Autodesk Inventor part; units mm, degrees
(part 2 of 3)
  line L407 (-50.8399, 107.9096) -> (-50.0992, 107.9096) construction
  line L408 (-50.0992, 107.9096) -> (-49.4855, 107.2111) construction
  line L409 (-49.4855, 107.2111) -> (-49.4855, 106.0543) construction
  line L410 (-49.4855, 106.0543) -> (-49.4855, 105.3065) construction
  line L411 (-49.4855, 105.3065) -> (-49.7183, 104.6082) construction
  line L412 (-49.7183, 104.6082) -> (-49.9582, 104.2413) construction
  line L413 (-49.9582, 104.2413) -> (-50.0569, 104.1002) construction
  line L414 (-50.0569, 104.1002) -> (-50.1839, 104.0649) construction
  line L415 (-50.1839, 104.0649) -> (-50.2756, 104.0649) construction
  line L416 (-50.2756, 104.0649) -> (-50.4802, 104.0649) construction
  line L417 (-50.4802, 104.0649) -> (-50.6777, 104.2201) construction
  line L418 (-50.6777, 104.2201) -> (-50.6777, 104.4247) construction
  line L419 (-50.6777, 104.4247) -> (-50.6777, 104.5234) construction
  line L420 (-50.6777, 104.5234) -> (-50.6354, 104.6221) construction
  line L421 (-50.6354, 104.6221) -> (-50.5859, 104.721) construction
  line L422 (-50.5859, 104.721) -> (-50.3884, 105.116) construction
  line L423 (-50.3884, 105.116) -> (-50.2403, 105.5957) construction
  line L424 (-50.2403, 105.5957) -> (-50.2403, 106.0966) construction
  line L425 (-50.2403, 106.0966) -> (-50.2403, 106.7385) construction
  line L426 (-50.2403, 106.7385) -> (-50.4731, 107.0842) construction
  line L427 (-50.4731, 107.0842) -> (-50.8258, 107.0842) construction
  line L428 (-50.8258, 107.0842) -> (-51.2138, 107.0842) construction
  line L429 (-51.2138, 107.0842) -> (-51.3126, 106.7104) construction
  line L430 (-51.3126, 106.7104) -> (-51.4819, 105.8567) construction
  line L431 (-51.4819, 105.8567) -> (-51.6512, 104.9961) construction
  line L432 (-51.6512, 104.9961) -> (-51.8417, 104.1636) construction
  line L433 (-51.8417, 104.1636) -> (-52.8786, 104.1636) construction
  line L434 (-52.8786, 104.1636) -> (-53.5982, 104.1636) construction
  line L435 (-53.5982, 104.1636) -> (-54.2895, 104.8197) construction
  line L436 (-54.2895, 104.8197) -> (-54.2895, 106.0755) construction
  line L437 (-54.2895, 106.0755) -> (-54.2895, 106.7033) construction
  line L438 (-54.2895, 106.7033) -> (-54.0638, 107.2959) construction
  line L439 (-54.0638, 107.2959) -> (-53.9156, 107.5427) construction
  line L440 (-44.8705, 56.7364) -> (-43.6289, 56.7364)
  line L441 (-43.6289, 56.7364) -> (-43.6289, 58.4153)
  spline S53 degree 3 poles (-43.6289, 58.4153) (-43.6289, 58.6481) (-43.4878, 58.7892) (-43.2692, 58.7892) (-43.0505, 58.7892) (-42.9094, 58.6481) (-42.9094, 58.4153) knots 2 2 2 2 3 3 3 4 4 4 4
  line L442 (-43.6289, 58.4153) -> (-43.6289, 58.6481) construction
  line L443 (-43.6289, 58.6481) -> (-43.4878, 58.7892) construction
  line L444 (-43.4878, 58.7892) -> (-43.2692, 58.7892) construction
  line L445 (-43.2692, 58.7892) -> (-43.0505, 58.7892) construction
  line L446 (-43.0505, 58.7892) -> (-42.9094, 58.6481) construction
  line L447 (-42.9094, 58.6481) -> (-42.9094, 58.4153) construction
  line L448 (-42.9094, 58.4153) -> (-42.9094, 56.7364)
  line L449 (-42.9094, 56.7364) -> (-41.3997, 56.7364)
  spline S54 degree 3 poles (-41.3997, 56.7364) (-41.1881, 56.7364) (-41.0541, 56.5742) (-41.0541, 56.3484) (-41.0541, 56.1227) (-41.1881, 55.9604) (-41.3997, 55.9604) knots 6 6 6 6 7 7 7 8 8 8 8
  line L450 (-41.3997, 56.7364) -> (-41.1881, 56.7364) construction
  line L451 (-41.1881, 56.7364) -> (-41.0541, 56.5742) construction
  line L452 (-41.0541, 56.5742) -> (-41.0541, 56.3484) construction
  line L453 (-41.0541, 56.3484) -> (-41.0541, 56.1227) construction
  line L454 (-41.0541, 56.1227) -> (-41.1881, 55.9604) construction
  line L455 (-41.1881, 55.9604) -> (-41.3997, 55.9604) construction
  line L456 (-41.3997, 55.9604) -> (-45.4137, 55.9604)
  spline S55 degree 3 poles (-45.4137, 55.9604) (-45.6183, 55.9604) (-45.7452, 56.0874) (-45.7452, 56.3131) knots 9 9 9 9 10 10 10 10
  line L457 (-45.4137, 55.9604) -> (-45.6183, 55.9604) construction
  line L458 (-45.6183, 55.9604) -> (-45.7452, 56.0874) construction
  line L459 (-45.7452, 56.0874) -> (-45.7452, 56.3131) construction
  line L460 (-45.7452, 56.3131) -> (-45.7452, 59.0008)
  spline S56 degree 3 poles (-45.7452, 59.0008) (-45.7452, 59.2336) (-45.6112, 59.3748) (-45.3855, 59.3748) (-45.1668, 59.3748) (-45.0328, 59.2336) (-45.0328, 59.0079) knots 11 11 11 11 12 12 12 13 13 13 13
  line L461 (-45.7452, 59.0008) -> (-45.7452, 59.2336) construction
  line L462 (-45.7452, 59.2336) -> (-45.6112, 59.3748) construction
  line L463 (-45.6112, 59.3748) -> (-45.3855, 59.3748) construction
  line L464 (-45.3855, 59.3748) -> (-45.1668, 59.3748) construction
  line L465 (-45.1668, 59.3748) -> (-45.0328, 59.2336) construction
  line L466 (-45.0328, 59.2336) -> (-45.0328, 59.0079) construction
  line L467 (-45.0328, 59.0079) -> (-45.0328, 56.8775)
  spline S57 degree 3 poles (-45.0328, 56.8775) (-45.0328, 56.7787) (-44.9904, 56.7364) (-44.8705, 56.7364) knots 14 14 14 14 15 15 15 15
  line L468 (-45.0328, 56.8775) -> (-45.0328, 56.7787) construction
  line L469 (-45.0328, 56.7787) -> (-44.9904, 56.7364) construction
  line L470 (-44.9904, 56.7364) -> (-44.8705, 56.7364) construction
  spline S58 degree 3 poles (-43.4314, 59.714) (-44.8212, 59.714) (-45.8228, 60.7863) (-45.8228, 62.183) (-45.8228, 63.5798) (-44.8212, 64.6591) (-43.4314, 64.6591) (-42.0347, 64.6591) (-41.0259, 63.5798) (-41.0259, 62.183) (-41.0259, 60.7863) (-42.0347, 59.714) (-43.4314, 59.714) knots 0 0 0 0 1 1 1 2 2 2 3 3 3 4 4 4 4
  line L471 (-43.4314, 59.714) -> (-44.8212, 59.714) construction
  line L472 (-44.8212, 59.714) -> (-45.8228, 60.7863) construction
  line L473 (-45.8228, 60.7863) -> (-45.8228, 62.183) construction
  line L474 (-45.8228, 62.183) -> (-45.8228, 63.5798) construction
  line L475 (-45.8228, 63.5798) -> (-44.8212, 64.6591) construction
  line L476 (-44.8212, 64.6591) -> (-43.4314, 64.6591) construction
  line L477 (-43.4314, 64.6591) -> (-42.0347, 64.6591) construction
  line L478 (-42.0347, 64.6591) -> (-41.0259, 63.5798) construction
  line L479 (-41.0259, 63.5798) -> (-41.0259, 62.183) construction
  line L480 (-41.0259, 62.183) -> (-41.0259, 60.7863) construction
  line L481 (-41.0259, 60.7863) -> (-42.0347, 59.714) construction
  line L482 (-42.0347, 59.714) -> (-43.4314, 59.714) construction
  spline S59 degree 3 poles (-41.7878, 62.183) (-41.7878, 63.0507) (-42.4086, 63.8126) (-43.4244, 63.8126) (-44.4402, 63.8126) (-45.061, 63.0507) (-45.061, 62.183) (-45.061, 61.3224) (-44.4402, 60.5606) (-43.4244, 60.5606) (-42.4086, 60.5606) (-41.7878, 61.3224) (-41.7878, 62.183) knots 0 0 0 0 1 1 1 2 2 2 3 3 3 4 4 4 4
  line L483 (-41.7878, 62.183) -> (-41.7878, 63.0507) construction
  line L484 (-41.7878, 63.0507) -> (-42.4086, 63.8126) construction
  line L485 (-42.4086, 63.8126) -> (-43.4244, 63.8126) construction
  line L486 (-43.4244, 63.8126) -> (-44.4402, 63.8126) construction
  line L487 (-44.4402, 63.8126) -> (-45.061, 63.0507) construction
  line L488 (-45.061, 63.0507) -> (-45.061, 62.183) construction
  line L489 (-45.061, 62.183) -> (-45.061, 61.3224) construction
  line L490 (-45.061, 61.3224) -> (-44.4402, 60.5606) construction
  line L491 (-44.4402, 60.5606) -> (-43.4244, 60.5606) construction
  line L492 (-43.4244, 60.5606) -> (-42.4086, 60.5606) construction
  line L493 (-42.4086, 60.5606) -> (-41.7878, 61.3224) construction
  line L494 (-41.7878, 61.3224) -> (-41.7878, 62.183) construction
  line L495 (-42.8247, 68.1872) -> (-41.703, 69.3087)
  spline S60 degree 3 poles (-41.703, 69.3087) (-41.6184, 69.4005) (-41.5337, 69.4429) (-41.4279, 69.4429) (-41.2445, 69.4429) (-41.0541, 69.2736) (-41.0541, 69.0477) (-41.0541, 68.9208) (-41.1105, 68.8362) (-41.2023, 68.7515) knots 1 1 1 1 2 2 2 3 3 3 4 4 4 4
  line L496 (-41.703, 69.3087) -> (-41.6184, 69.4005) construction
  line L497 (-41.6184, 69.4005) -> (-41.5337, 69.4429) construction
  line L498 (-41.5337, 69.4429) -> (-41.4279, 69.4429) construction
  line L499 (-41.4279, 69.4429) -> (-41.2445, 69.4429) construction
  line L500 (-41.2445, 69.4429) -> (-41.0541, 69.2736) construction
  line L501 (-41.0541, 69.2736) -> (-41.0541, 69.0477) construction
  line L502 (-41.0541, 69.0477) -> (-41.0541, 68.9208) construction
  line L503 (-41.0541, 68.9208) -> (-41.1105, 68.8362) construction
  line L504 (-41.1105, 68.8362) -> (-41.2023, 68.7515) construction
  line L505 (-41.2023, 68.7515) -> (-42.719, 67.2983)
  line L506 (-42.719, 67.2983) -> (-42.719, 66.5083)
  line L507 (-42.719, 66.5083) -> (-41.3997, 66.5083)
  spline S61 degree 3 poles (-41.3997, 66.5083) (-41.1881, 66.5083) (-41.0541, 66.346) (-41.0541, 66.1203) (-41.0541, 65.8945) (-41.1881, 65.7323) (-41.3997, 65.7323) knots 7 7 7 7 8 8 8 9 9 9 9
  line L508 (-41.3997, 66.5083) -> (-41.1881, 66.5083) construction
  line L509 (-41.1881, 66.5083) -> (-41.0541, 66.346) construction
  line L510 (-41.0541, 66.346) -> (-41.0541, 66.1203) construction
  line L511 (-41.0541, 66.1203) -> (-41.0541, 65.8945) construction
  line L512 (-41.0541, 65.8945) -> (-41.1881, 65.7323) construction
  line L513 (-41.1881, 65.7323) -> (-41.3997, 65.7323) construction
  line L514 (-41.3997, 65.7323) -> (-45.4137, 65.7323)
  spline S62 degree 3 poles (-45.4137, 65.7323) (-45.6183, 65.7323) (-45.7452, 65.8592) (-45.7452, 66.085) knots 10 10 10 10 11 11 11 11
  line L515 (-45.4137, 65.7323) -> (-45.6183, 65.7323) construction
  line L516 (-45.6183, 65.7323) -> (-45.7452, 65.8592) construction
  line L517 (-45.7452, 65.8592) -> (-45.7452, 66.085) construction
  line L518 (-45.7452, 66.085) -> (-45.7452, 67.5381)
  spline S63 degree 3 poles (-45.7452, 67.5381) (-45.7452, 68.8362) (-45.0398, 69.3793) (-44.278, 69.3793) (-43.7065, 69.3793) (-43.0153, 69.0266) (-42.8247, 68.1872) knots 12 12 12 12 13 13 13 14 14 14 14
  line L519 (-45.7452, 67.5381) -> (-45.7452, 68.8362) construction
  line L520 (-45.7452, 68.8362) -> (-45.0398, 69.3793) construction
  line L521 (-45.0398, 69.3793) -> (-44.278, 69.3793) construction
  line L522 (-44.278, 69.3793) -> (-43.7065, 69.3793) construction
  line L523 (-43.7065, 69.3793) -> (-43.0153, 69.0266) construction
  line L524 (-43.0153, 69.0266) -> (-42.8247, 68.1872) construction
  spline S64 degree 3 poles (-43.4173, 67.4818) (-43.4173, 68.2576) (-43.7841, 68.5329) (-44.2285, 68.5329) (-44.666, 68.5329) (-45.0328, 68.2576) (-45.0328, 67.4818) knots 0 0 0 0 1 1 1 2 2 2 2
  line L525 (-43.4173, 67.4818) -> (-43.4173, 68.2576) construction
  line L526 (-43.4173, 68.2576) -> (-43.7841, 68.5329) construction
  line L527 (-43.7841, 68.5329) -> (-44.2285, 68.5329) construction
  line L528 (-44.2285, 68.5329) -> (-44.666, 68.5329) construction
  line L529 (-44.666, 68.5329) -> (-45.0328, 68.2576) construction
  line L530 (-45.0328, 68.2576) -> (-45.0328, 67.4818) construction
  line L531 (-45.0328, 67.4818) -> (-45.0328, 66.6493)
  spline S65 degree 3 poles (-45.0328, 66.6493) (-45.0328, 66.5506) (-44.9904, 66.5083) (-44.8705, 66.5083) knots 3 3 3 3 4 4 4 4
  line L532 (-45.0328, 66.6493) -> (-45.0328, 66.5506) construction
  line L533 (-45.0328, 66.5506) -> (-44.9904, 66.5083) construction
  line L534 (-44.9904, 66.5083) -> (-44.8705, 66.5083) construction
  line L535 (-44.8705, 66.5083) -> (-43.4173, 66.5083)
  line L536 (-43.4173, 66.5083) -> (-43.4173, 67.4818)
  line L537 (-44.546, 74.2405) -> (-43.0575, 73.2248)
  spline S66 degree 3 poles (-43.0575, 73.2248) (-42.8459, 73.0837) (-42.7613, 72.9707) (-42.7613, 72.7803) (-42.7613, 72.5969) (-42.8459, 72.4911) (-43.0575, 72.343) knots 1 1 1 1 2 2 2 3 3 3 3
  line L538 (-43.0575, 73.2248) -> (-42.8459, 73.0837) construction
  line L539 (-42.8459, 73.0837) -> (-42.7613, 72.9707) construction
  line L540 (-42.7613, 72.9707) -> (-42.7613, 72.7803) construction
  line L541 (-42.7613, 72.7803) -> (-42.7613, 72.5969) construction
  line L542 (-42.7613, 72.5969) -> (-42.8459, 72.4911) construction
  line L543 (-42.8459, 72.4911) -> (-43.0575, 72.343) construction
  line L544 (-43.0575, 72.343) -> (-44.546, 71.327)
  line L545 (-44.546, 71.327) -> (-44.546, 71.306)
  line L546 (-44.546, 71.306) -> (-41.3997, 71.306)
  spline S67 degree 3 poles (-41.3997, 71.306) (-41.1881, 71.306) (-41.0541, 71.1437) (-41.0541, 70.9179) (-41.0541, 70.6923) (-41.1881, 70.53) (-41.3997, 70.53) knots 6 6 6 6 7 7 7 8 8 8 8
  line L547 (-41.3997, 71.306) -> (-41.1881, 71.306) construction
  line L548 (-41.1881, 71.306) -> (-41.0541, 71.1437) construction
  line L549 (-41.0541, 71.1437) -> (-41.0541, 70.9179) construction
  line L550 (-41.0541, 70.9179) -> (-41.0541, 70.6923) construction
  line L551 (-41.0541, 70.6923) -> (-41.1881, 70.53) construction
  line L552 (-41.1881, 70.53) -> (-41.3997, 70.53) construction
  line L553 (-41.3997, 70.53) -> (-45.3361, 70.53)
  spline S68 degree 3 poles (-45.3361, 70.53) (-45.6112, 70.53) (-45.7876, 70.7274) (-45.7876, 70.9885) knots 9 9 9 9 10 10 10 10
  line L554 (-45.3361, 70.53) -> (-45.6112, 70.53) construction
  line L555 (-45.6112, 70.53) -> (-45.7876, 70.7274) construction
  line L556 (-45.7876, 70.7274) -> (-45.7876, 70.9885) construction
  line L557 (-45.7876, 70.9885) -> (-45.7876, 71.0449)
  spline S69 degree 3 poles (-45.7876, 71.0449) (-45.7876, 71.3131) (-45.6253, 71.4822) (-45.4137, 71.6233) knots 11 11 11 11 12 12 12 12
  line L558 (-45.7876, 71.0449) -> (-45.7876, 71.3131) construction
  line L559 (-45.7876, 71.3131) -> (-45.6253, 71.4822) construction
  line L560 (-45.6253, 71.4822) -> (-45.4137, 71.6233) construction
  line L561 (-45.4137, 71.6233) -> (-43.6925, 72.8015)
  line L562 (-43.6925, 72.8015) -> (-43.6925, 72.8086)
  line L563 (-43.6925, 72.8086) -> (-45.4208, 73.9796)
  spline S70 degree 3 poles (-45.4208, 73.9796) (-45.6253, 74.1206) (-45.7876, 74.2547) (-45.7876, 74.5227) knots 15 15 15 15 16 16 16 16
  line L564 (-45.4208, 73.9796) -> (-45.6253, 74.1206) construction
  line L565 (-45.6253, 74.1206) -> (-45.7876, 74.2547) construction
  line L566 (-45.7876, 74.2547) -> (-45.7876, 74.5227) construction
  line L567 (-45.7876, 74.5227) -> (-45.7876, 74.5792)
  spline S71 degree 3 poles (-45.7876, 74.5792) (-45.7876, 74.8331) (-45.6112, 75.0307) (-45.3361, 75.0307) knots 17 17 17 17 18 18 18 18
  line L568 (-45.7876, 74.5792) -> (-45.7876, 74.8331) construction
  line L569 (-45.7876, 74.8331) -> (-45.6112, 75.0307) construction
  line L570 (-45.6112, 75.0307) -> (-45.3361, 75.0307) construction
  line L571 (-45.3361, 75.0307) -> (-41.3997, 75.0307)
  spline S72 degree 3 poles (-41.3997, 75.0307) (-41.1881, 75.0307) (-41.0541, 74.8684) (-41.0541, 74.6426) (-41.0541, 74.4169) (-41.1881, 74.2547) (-41.3997, 74.2547) knots 19 19 19 19 20 20 20 21 21 21 21
  line L572 (-41.3997, 75.0307) -> (-41.1881, 75.0307) construction
  line L573 (-41.1881, 75.0307) -> (-41.0541, 74.8684) construction
  line L574 (-41.0541, 74.8684) -> (-41.0541, 74.6426) construction
  line L575 (-41.0541, 74.6426) -> (-41.0541, 74.4169) construction
  line L576 (-41.0541, 74.4169) -> (-41.1881, 74.2547) construction
  line L577 (-41.1881, 74.2547) -> (-41.3997, 74.2547) construction
  line L578 (-41.3997, 74.2547) -> (-44.546, 74.2547)
  line L579 (-44.546, 74.2547) -> (-44.546, 74.2405)
  spline S73 degree 3 poles (-41.7666, 78.3612) (-41.7666, 79.116) (-42.2815, 79.5887) (-43.0858, 79.5887) knots 0 0 0 0 1 1 1 1
  line L580 (-41.7666, 78.3612) -> (-41.7666, 79.116) construction
  line L581 (-41.7666, 79.116) -> (-42.2815, 79.5887) construction
  line L582 (-42.2815, 79.5887) -> (-43.0858, 79.5887) construction
  line L583 (-43.0858, 79.5887) -> (-45.449, 79.5887)
  spline S74 degree 3 poles (-45.449, 79.5887) (-45.6536, 79.5887) (-45.7947, 79.7508) (-45.7947, 79.9766) (-45.7947, 80.2023) (-45.6536, 80.3645) (-45.449, 80.3645) knots 2 2 2 2 3 3 3 4 4 4 4
  line L584 (-45.449, 79.5887) -> (-45.6536, 79.5887) construction
  line L585 (-45.6536, 79.5887) -> (-45.7947, 79.7508) construction
  line L586 (-45.7947, 79.7508) -> (-45.7947, 79.9766) construction
  line L587 (-45.7947, 79.9766) -> (-45.7947, 80.2023) construction
  line L588 (-45.7947, 80.2023) -> (-45.6536, 80.3645) construction
  line L589 (-45.6536, 80.3645) -> (-45.449, 80.3645) construction
  line L590 (-45.449, 80.3645) -> (-43.0434, 80.3645)
  spline S75 degree 3 poles (-43.0434, 80.3645) (-41.8723, 80.3645) (-41.0118, 79.6168) (-41.0118, 78.3612) (-41.0118, 77.0984) (-41.8723, 76.3577) (-43.0434, 76.3577) knots 5 5 5 5 6 6 6 7 7 7 7
  line L591 (-43.0434, 80.3645) -> (-41.8723, 80.3645) construction
  line L592 (-41.8723, 80.3645) -> (-41.0118, 79.6168) construction
  line L593 (-41.0118, 79.6168) -> (-41.0118, 78.3612) construction
  line L594 (-41.0118, 78.3612) -> (-41.0118, 77.0984) construction
  line L595 (-41.0118, 77.0984) -> (-41.8723, 76.3577) construction
  line L596 (-41.8723, 76.3577) -> (-43.0434, 76.3577) construction
  line L597 (-43.0434, 76.3577) -> (-45.449, 76.3577)
  spline S76 degree 3 poles (-45.449, 76.3577) (-45.6536, 76.3577) (-45.7947, 76.52) (-45.7947, 76.7456) (-45.7947, 76.9715) (-45.6536, 77.1337) (-45.449, 77.1337) knots 8 8 8 8 9 9 9 10 10 10 10
  line L598 (-45.449, 76.3577) -> (-45.6536, 76.3577) construction
  line L599 (-45.6536, 76.3577) -> (-45.7947, 76.52) construction
  line L600 (-45.7947, 76.52) -> (-45.7947, 76.7456) construction
  line L601 (-45.7947, 76.7456) -> (-45.7947, 76.9715) construction
  line L602 (-45.7947, 76.9715) -> (-45.6536, 77.1337) construction
  line L603 (-45.6536, 77.1337) -> (-45.449, 77.1337) construction
  line L604 (-45.449, 77.1337) -> (-43.0858, 77.1337)
  spline S77 degree 3 poles (-43.0858, 77.1337) (-42.2886, 77.1337) (-41.7666, 77.5993) (-41.7666, 78.3612) knots 11 11 11 11 12 12 12 12
  line L605 (-43.0858, 77.1337) -> (-42.2886, 77.1337) construction
  line L606 (-42.2886, 77.1337) -> (-41.7666, 77.5993) construction
  line L607 (-41.7666, 77.5993) -> (-41.7666, 78.3612) construction
  spline S78 degree 3 poles (-45.7876, 82.0797) (-45.7876, 82.3055) (-45.6536, 82.4678) (-45.449, 82.4678) knots 0 0 0 0 1 1 1 1
  line L608 (-45.7876, 82.0797) -> (-45.7876, 82.3055) construction
  line L609 (-45.7876, 82.3055) -> (-45.6536, 82.4678) construction
  line L610 (-45.6536, 82.4678) -> (-45.449, 82.4678) construction
  line L611 (-45.449, 82.4678) -> (-41.9853, 82.4678)
  spline S79 degree 3 poles (-41.9853, 82.4678) (-41.8582, 82.4678) (-41.8229, 82.51) (-41.8229, 82.6088) knots 2 2 2 2 3 3 3 3
  line L612 (-41.9853, 82.4678) -> (-41.8582, 82.4678) construction
  line L613 (-41.8582, 82.4678) -> (-41.8229, 82.51) construction
  line L614 (-41.8229, 82.51) -> (-41.8229, 82.6088) construction
  line L615 (-41.8229, 82.6088) -> (-41.8229, 84.6687)
  spline S80 degree 3 poles (-41.8229, 84.6687) (-41.8229, 84.9014) (-41.6889, 85.0425) (-41.4632, 85.0425) (-41.2374, 85.0425) (-41.1034, 84.9014) (-41.1034, 84.6687) knots 4 4 4 4 5 5 5 6 6 6 6
  line L616 (-41.8229, 84.6687) -> (-41.8229, 84.9014) construction
  line L617 (-41.8229, 84.9014) -> (-41.6889, 85.0425) construction
  line L618 (-41.6889, 85.0425) -> (-41.4632, 85.0425) construction
  line L619 (-41.4632, 85.0425) -> (-41.2374, 85.0425) construction
  line L620 (-41.2374, 85.0425) -> (-41.1034, 84.9014) construction
  line L621 (-41.1034, 84.9014) -> (-41.1034, 84.6687) construction
  line L622 (-41.1034, 84.6687) -> (-41.1034, 82.0726)
  spline S81 degree 3 poles (-41.1034, 82.0726) (-41.1034, 81.8399) (-41.2303, 81.6918) (-41.4632, 81.6918) knots 7 7 7 7 8 8 8 8
  line L623 (-41.1034, 82.0726) -> (-41.1034, 81.8399) construction
  line L624 (-41.1034, 81.8399) -> (-41.2303, 81.6918) construction
  line L625 (-41.2303, 81.6918) -> (-41.4632, 81.6918) construction
  line L626 (-41.4632, 81.6918) -> (-45.449, 81.6918)
  spline S82 degree 3 poles (-45.449, 81.6918) (-45.6536, 81.6918) (-45.7876, 81.854) (-45.7876, 82.0797) knots 9 9 9 9 10 10 10 10
  line L627 (-45.449, 81.6918) -> (-45.6536, 81.6918) construction
  line L628 (-45.6536, 81.6918) -> (-45.7876, 81.854) construction
  line L629 (-45.7876, 81.854) -> (-45.7876, 82.0797) construction
  line L630 (-42.2392, 86.6162) -> (-41.3433, 86.2495)
  spline S83 degree 3 poles (-41.3433, 86.2495) (-41.1528, 86.1718) (-41.0541, 86.0519) (-41.0541, 85.8684) (-41.0541, 85.6428) (-41.2023, 85.4876) (-41.4067, 85.4734) knots 1 1 1 1 2 2 2 3 3 3 3
  line L631 (-41.3433, 86.2495) -> (-41.1528, 86.1718) construction
  line L632 (-41.1528, 86.1718) -> (-41.0541, 86.0519) construction
  line L633 (-41.0541, 86.0519) -> (-41.0541, 85.8684) construction
  line L634 (-41.0541, 85.8684) -> (-41.0541, 85.6428) construction
  line L635 (-41.0541, 85.6428) -> (-41.2023, 85.4876) construction
  line L636 (-41.2023, 85.4876) -> (-41.4067, 85.4734) construction
  spline S84 degree 3 poles (-41.4067, 85.4734) (-41.4986, 85.4664) (-41.5831, 85.4946) (-41.6818, 85.537) knots 3 3 3 3 4 4 4 4
  line L637 (-41.4067, 85.4734) -> (-41.4986, 85.4664) construction
  line L638 (-41.4986, 85.4664) -> (-41.5831, 85.4946) construction
  line L639 (-41.5831, 85.4946) -> (-41.6818, 85.537) construction
  line L640 (-41.6818, 85.537) -> (-45.2444, 87.0184)
  spline S85 degree 3 poles (-45.2444, 87.0184) (-45.6395, 87.1736) (-45.7876, 87.3851) (-45.7876, 87.7026) knots 5 5 5 5 6 6 6 6
  line L641 (-45.2444, 87.0184) -> (-45.6395, 87.1736) construction
  line L642 (-45.6395, 87.1736) -> (-45.7876, 87.3851) construction
  line L643 (-45.7876, 87.3851) -> (-45.7876, 87.7026) construction
  line L644 (-45.7876, 87.7026) -> (-45.7876, 87.752)
  spline S86 degree 3 poles (-45.7876, 87.752) (-45.7876, 88.0766) (-45.6395, 88.281) (-45.2444, 88.4433) knots 7 7 7 7 8 8 8 8
  line L645 (-45.7876, 87.752) -> (-45.7876, 88.0766) construction
  line L646 (-45.7876, 88.0766) -> (-45.6395, 88.281) construction
  line L647 (-45.6395, 88.281) -> (-45.2444, 88.4433) construction
  line L648 (-45.2444, 88.4433) -> (-41.6538, 89.9247)
  spline S87 degree 3 poles (-41.6538, 89.9247) (-41.5619, 89.96) (-41.4844, 89.9812) (-41.4279, 89.9812) (-41.2093, 89.9812) (-41.0541, 89.8048) (-41.0541, 89.5721) (-41.0541, 89.4027) (-41.1599, 89.2617) (-41.3504, 89.184) knots 9 9 9 9 10 10 10 11 11 11 12 12 12 12
  line L649 (-41.6538, 89.9247) -> (-41.5619, 89.96) construction
  line L650 (-41.5619, 89.96) -> (-41.4844, 89.9812) construction
  line L651 (-41.4844, 89.9812) -> (-41.4279, 89.9812) construction
  line L652 (-41.4279, 89.9812) -> (-41.2093, 89.9812) construction
  line L653 (-41.2093, 89.9812) -> (-41.0541, 89.8048) construction
  line L654 (-41.0541, 89.8048) -> (-41.0541, 89.5721) construction
  line L655 (-41.0541, 89.5721) -> (-41.0541, 89.4027) construction
  line L656 (-41.0541, 89.4027) -> (-41.1599, 89.2617) construction
  line L657 (-41.1599, 89.2617) -> (-41.3504, 89.184) construction
  line L658 (-41.3504, 89.184) -> (-42.2392, 88.8243)
  line L659 (-42.2392, 88.8243) -> (-42.2392, 86.6162)
  line L660 (-42.9447, 88.5492) -> (-45.0116, 87.7379)
  line L661 (-45.0116, 87.7379) -> (-45.0116, 87.7167)
  line L662 (-45.0116, 87.7167) -> (-42.9447, 86.8844)
  line L663 (-42.9447, 86.8844) -> (-42.9447, 88.5492)
  spline S88 degree 3 poles (-45.3855, 89.8479) (-45.6112, 89.8479) (-45.7452, 89.996) (-45.7452, 90.2289) knots 0 0 0 0 1 1 1 1
  line L664 (-45.3855, 89.8479) -> (-45.6112, 89.8479) construction
  line L665 (-45.6112, 89.8479) -> (-45.7452, 89.996) construction
  line L666 (-45.7452, 89.996) -> (-45.7452, 90.2289) construction
  line L667 (-45.7452, 90.2289) -> (-45.7452, 93.8337)
  spline S89 degree 3 poles (-45.7452, 93.8337) (-45.7452, 94.0664) (-45.6112, 94.2075) (-45.3855, 94.2075) (-45.1668, 94.2075) (-45.0328, 94.0664) (-45.0328, 93.8337) knots 2 2 2 2 3 3 3 4 4 4 4
  line L668 (-45.7452, 93.8337) -> (-45.7452, 94.0664) construction
  line L669 (-45.7452, 94.0664) -> (-45.6112, 94.2075) construction
  line L670 (-45.6112, 94.2075) -> (-45.3855, 94.2075) construction
  line L671 (-45.3855, 94.2075) -> (-45.1668, 94.2075) construction
  line L672 (-45.1668, 94.2075) -> (-45.0328, 94.0664) construction
  line L673 (-45.0328, 94.0664) -> (-45.0328, 93.8337) construction
  line L674 (-45.0328, 93.8337) -> (-45.0328, 92.4227)
  line L675 (-45.0328, 92.4227) -> (-41.3997, 92.4227)
  spline S90 degree 3 poles (-41.3997, 92.4227) (-41.1952, 92.4227) (-41.0541, 92.2605) (-41.0541, 92.0348) (-41.0541, 91.809) (-41.1952, 91.6467) (-41.3997, 91.6467) knots 6 6 6 6 7 7 7 8 8 8 8
  line L676 (-41.3997, 92.4227) -> (-41.1952, 92.4227) construction
  line L677 (-41.1952, 92.4227) -> (-41.0541, 92.2605) construction
  line L678 (-41.0541, 92.2605) -> (-41.0541, 92.0348) construction
  line L679 (-41.0541, 92.0348) -> (-41.0541, 91.809) construction
  line L680 (-41.0541, 91.809) -> (-41.1952, 91.6467) construction
  line L681 (-41.1952, 91.6467) -> (-41.3997, 91.6467) construction
  line L682 (-41.3997, 91.6467) -> (-45.0328, 91.6467)
  line L683 (-45.0328, 91.6467) -> (-45.0328, 90.2218)
  spline S91 degree 3 poles (-45.0328, 90.2218) (-45.0328, 89.996) (-45.1668, 89.8479) (-45.3855, 89.8479) knots 10 10 10 10 11 11 11 11
  line L684 (-45.0328, 90.2218) -> (-45.0328, 89.996) construction
  line L685 (-45.0328, 89.996) -> (-45.1668, 89.8479) construction
  line L686 (-45.1668, 89.8479) -> (-45.3855, 89.8479) construction
  spline S92 degree 3 poles (-45.7947, 95.3864) (-45.7947, 95.612) (-45.6536, 95.7743) (-45.449, 95.7743) knots 0 0 0 0 1 1 1 1
  line L687 (-45.7947, 95.3864) -> (-45.7947, 95.612) construction
  line L688 (-45.7947, 95.612) -> (-45.6536, 95.7743) construction
  line L689 (-45.6536, 95.7743) -> (-45.449, 95.7743) construction
  line L690 (-45.449, 95.7743) -> (-41.3997, 95.7743)
  spline S93 degree 3 poles (-41.3997, 95.7743) (-41.1952, 95.7743) (-41.0541, 95.612) (-41.0541, 95.3864) (-41.0541, 95.1605) (-41.1952, 94.9983) (-41.3997, 94.9983) knots 2 2 2 2 3 3 3 4 4 4 4
  line L691 (-41.3997, 95.7743) -> (-41.1952, 95.7743) construction
  line L692 (-41.1952, 95.7743) -> (-41.0541, 95.612) construction
  line L693 (-41.0541, 95.612) -> (-41.0541, 95.3864) construction
  line L694 (-41.0541, 95.3864) -> (-41.0541, 95.1605) construction
  line L695 (-41.0541, 95.1605) -> (-41.1952, 94.9983) construction
  line L696 (-41.1952, 94.9983) -> (-41.3997, 94.9983) construction
  line L697 (-41.3997, 94.9983) -> (-45.449, 94.9983)
  spline S94 degree 3 poles (-45.449, 94.9983) (-45.6536, 94.9983) (-45.7947, 95.1605) (-45.7947, 95.3864) knots 5 5 5 5 6 6 6 6
  line L698 (-45.449, 94.9983) -> (-45.6536, 94.9983) construction
  line L699 (-45.6536, 94.9983) -> (-45.7947, 95.1605) construction
  line L700 (-45.7947, 95.1605) -> (-45.7947, 95.3864) construction
  spline S95 degree 3 poles (-43.4314, 96.8398) (-44.8212, 96.8398) (-45.8228, 97.9121) (-45.8228, 99.3089) (-45.8228, 100.7058) (-44.8212, 101.7851) (-43.4314, 101.7851) (-42.0347, 101.7851) (-41.0259, 100.7058) (-41.0259, 99.3089) (-41.0259, 97.9121) (-42.0347, 96.8398) (-43.4314, 96.8398) knots 0 0 0 0 1 1 1 2 2 2 3 3 3 4 4 4 4
  line L701 (-43.4314, 96.8398) -> (-44.8212, 96.8398) construction
  line L702 (-44.8212, 96.8398) -> (-45.8228, 97.9121) construction
  line L703 (-45.8228, 97.9121) -> (-45.8228, 99.3089) construction
  line L704 (-45.8228, 99.3089) -> (-45.8228, 100.7058) construction
  line L705 (-45.8228, 100.7058) -> (-44.8212, 101.7851) construction
  line L706 (-44.8212, 101.7851) -> (-43.4314, 101.7851) construction
  line L707 (-43.4314, 101.7851) -> (-42.0347, 101.7851) construction
  line L708 (-42.0347, 101.7851) -> (-41.0259, 100.7058) construction
  line L709 (-41.0259, 100.7058) -> (-41.0259, 99.3089) construction
  line L710 (-41.0259, 99.3089) -> (-41.0259, 97.9121) construction
  line L711 (-41.0259, 97.9121) -> (-42.0347, 96.8398) construction
  line L712 (-42.0347, 96.8398) -> (-43.4314, 96.8398) construction
  spline S96 degree 3 poles (-41.7878, 99.3089) (-41.7878, 100.1766) (-42.4086, 100.9385) (-43.4244, 100.9385) (-44.4402, 100.9385) (-45.061, 100.1766) (-45.061, 99.3089) (-45.061, 98.4484) (-44.4402, 97.6865) (-43.4244, 97.6865) (-42.4086, 97.6865) (-41.7878, 98.4484) (-41.7878, 99.3089) knots 0 0 0 0 1 1 1 2 2 2 3 3 3 4 4 4 4
  line L713 (-41.7878, 99.3089) -> (-41.7878, 100.1766) construction
  line L714 (-41.7878, 100.1766) -> (-42.4086, 100.9385) construction
  line L715 (-42.4086, 100.9385) -> (-43.4244, 100.9385) construction
  line L716 (-43.4244, 100.9385) -> (-44.4402, 100.9385) construction
  line L717 (-44.4402, 100.9385) -> (-45.061, 100.1766) construction
  line L718 (-45.061, 100.1766) -> (-45.061, 99.3089) construction
  line L719 (-45.061, 99.3089) -> (-45.061, 98.4484) construction
  line L720 (-45.061, 98.4484) -> (-44.4402, 97.6865) construction
  line L721 (-44.4402, 97.6865) -> (-43.4244, 97.6865) construction
  line L722 (-43.4244, 97.6865) -> (-42.4086, 97.6865) construction
  line L723 (-42.4086, 97.6865) -> (-41.7878, 98.4484) construction
  line L724 (-41.7878, 98.4484) -> (-41.7878, 99.3089) construction
  line L725 (-41.0541, 106.484) -> (-41.0541, 106.456)
  spline S97 degree 3 poles (-41.0541, 106.456) (-41.0541, 106.216) (-41.1599, 106.0608) (-41.4067, 105.8844) knots 1 1 1 1 2 2 2 2
  line L726 (-41.0541, 106.456) -> (-41.0541, 106.216) construction
  line L727 (-41.0541, 106.216) -> (-41.1599, 106.0608) construction
  line L728 (-41.1599, 106.0608) -> (-41.4067, 105.8844) construction
  line L729 (-41.4067, 105.8844) -> (-44.5601, 103.6341)
  line L730 (-44.5601, 103.6341) -> (-41.3997, 103.6341)
  spline S98 degree 3 poles (-41.3997, 103.6341) (-41.1952, 103.6341) (-41.0541, 103.4718) (-41.0541, 103.2462) (-41.0541, 103.0204) (-41.1952, 102.8581) (-41.3997, 102.8581) knots 4 4 4 4 5 5 5 6 6 6 6
  line L731 (-41.3997, 103.6341) -> (-41.1952, 103.6341) construction
  line L732 (-41.1952, 103.6341) -> (-41.0541, 103.4718) construction
  line L733 (-41.0541, 103.4718) -> (-41.0541, 103.2462) construction
  line L734 (-41.0541, 103.2462) -> (-41.0541, 103.0204) construction
  line L735 (-41.0541, 103.0204) -> (-41.1952, 102.8581) construction
  line L736 (-41.1952, 102.8581) -> (-41.3997, 102.8581) construction
  line L737 (-41.3997, 102.8581) -> (-45.322, 102.8581)
  spline S99 degree 3 poles (-45.322, 102.8581) (-45.6042, 102.8581) (-45.7876, 103.0486) (-45.7876, 103.2886) knots 7 7 7 7 8 8 8 8
  line L738 (-45.322, 102.8581) -> (-45.6042, 102.8581) construction
  line L739 (-45.6042, 102.8581) -> (-45.7876, 103.0486) construction
  line L740 (-45.7876, 103.0486) -> (-45.7876, 103.2886) construction
  line L741 (-45.7876, 103.2886) -> (-45.7876, 103.3308)
  spline S100 degree 3 poles (-45.7876, 103.3308) (-45.7876, 103.5707) (-45.7029, 103.6977) (-45.3996, 103.9233) knots 9 9 9 9 10 10 10 10
  line L742 (-45.7876, 103.3308) -> (-45.7876, 103.5707) construction
  line L743 (-45.7876, 103.5707) -> (-45.7029, 103.6977) construction
  line L744 (-45.7029, 103.6977) -> (-45.3996, 103.9233) construction
  line L745 (-45.3996, 103.9233) -> (-42.338, 106.1736)
  line L746 (-42.338, 106.1736) -> (-45.449, 106.1736)
  spline S101 degree 3 poles (-45.449, 106.1736) (-45.6536, 106.1736) (-45.7947, 106.3359) (-45.7947, 106.5617) (-45.7947, 106.7874) (-45.6536, 106.9497) (-45.449, 106.9497) knots 12 12 12 12 13 13 13 14 14 14 14
  line L747 (-45.449, 106.1736) -> (-45.6536, 106.1736) construction
  line L748 (-45.6536, 106.1736) -> (-45.7947, 106.3359) construction
  line L749 (-45.7947, 106.3359) -> (-45.7947, 106.5617) construction
  line L750 (-45.7947, 106.5617) -> (-45.7947, 106.7874) construction
  line L751 (-45.7947, 106.7874) -> (-45.6536, 106.9497) construction
  line L752 (-45.6536, 106.9497) -> (-45.449, 106.9497) construction
  line L753 (-45.449, 106.9497) -> (-41.4703, 106.9497)
  spline S102 degree 3 poles (-41.4703, 106.9497) (-41.2233, 106.9497) (-41.0541, 106.7311) (-41.0541, 106.484) knots 15 15 15 15 16 16 16 16
  line L754 (-41.4703, 106.9497) -> (-41.2233, 106.9497) construction
  line L755 (-41.2233, 106.9497) -> (-41.0541, 106.7311) construction
  line L756 (-41.0541, 106.7311) -> (-41.0541, 106.484) construction
  spline S103 degree 3 poles (-37.3209, 56.3484) (-37.3209, 56.5742) (-37.1868, 56.7364) (-36.9822, 56.7364) knots 0 0 0 0 1 1 1 1
  line L757 (-37.3209, 56.3484) -> (-37.3209, 56.5742) construction
  line L758 (-37.3209, 56.5742) -> (-37.1868, 56.7364) construction
  line L759 (-37.1868, 56.7364) -> (-36.9822, 56.7364) construction
  line L760 (-36.9822, 56.7364) -> (-33.5185, 56.7364)
  spline S104 degree 3 poles (-33.5185, 56.7364) (-33.3916, 56.7364) (-33.3562, 56.7787) (-33.3562, 56.8775) knots 2 2 2 2 3 3 3 3
  line L761 (-33.5185, 56.7364) -> (-33.3916, 56.7364) construction
  line L762 (-33.3916, 56.7364) -> (-33.3562, 56.7787) construction
  line L763 (-33.3562, 56.7787) -> (-33.3562, 56.8775) construction
  line L764 (-33.3562, 56.8775) -> (-33.3562, 58.9373)
  spline S105 degree 3 poles (-33.3562, 58.9373) (-33.3562, 59.1701) (-33.2222, 59.3112) (-32.9966, 59.3112) (-32.7707, 59.3112) (-32.6367, 59.1701) (-32.6367, 58.9373) knots 4 4 4 4 5 5 5 6 6 6 6
  line L765 (-33.3562, 58.9373) -> (-33.3562, 59.1701) construction
  line L766 (-33.3562, 59.1701) -> (-33.2222, 59.3112) construction
  line L767 (-33.2222, 59.3112) -> (-32.9966, 59.3112) construction
  line L768 (-32.9966, 59.3112) -> (-32.7707, 59.3112) construction
  line L769 (-32.7707, 59.3112) -> (-32.6367, 59.1701) construction
  line L770 (-32.6367, 59.1701) -> (-32.6367, 58.9373) construction
  line L771 (-32.6367, 58.9373) -> (-32.6367, 56.3414)
  spline S106 degree 3 poles (-32.6367, 56.3414) (-32.6367, 56.1086) (-32.7637, 55.9604) (-32.9966, 55.9604) knots 7 7 7 7 8 8 8 8
  line L772 (-32.6367, 56.3414) -> (-32.6367, 56.1086) construction
  line L773 (-32.6367, 56.1086) -> (-32.7637, 55.9604) construction
  line L774 (-32.7637, 55.9604) -> (-32.9966, 55.9604) construction
  line L775 (-32.9966, 55.9604) -> (-36.9822, 55.9604)
  spline S107 degree 3 poles (-36.9822, 55.9604) (-37.1868, 55.9604) (-37.3209, 56.1227) (-37.3209, 56.3484) knots 9 9 9 9 10 10 10 10
  line L776 (-36.9822, 55.9604) -> (-37.1868, 55.9604) construction
  line L777 (-37.1868, 55.9604) -> (-37.3209, 56.1227) construction
  line L778 (-37.3209, 56.1227) -> (-37.3209, 56.3484) construction
  line L779 (-33.7726, 60.8849) -> (-32.8767, 60.5181)
  spline S108 degree 3 poles (-32.8767, 60.5181) (-32.6862, 60.4405) (-32.5873, 60.3206) (-32.5873, 60.1372) (-32.5873, 59.9114) (-32.7356, 59.7562) (-32.9401, 59.7421) knots 1 1 1 1 2 2 2 3 3 3 3
  line L780 (-32.8767, 60.5181) -> (-32.6862, 60.4405) construction
  line L781 (-32.6862, 60.4405) -> (-32.5873, 60.3206) construction
  line L782 (-32.5873, 60.3206) -> (-32.5873, 60.1372) construction
  line L783 (-32.5873, 60.1372) -> (-32.5873, 59.9114) construction
  line L784 (-32.5873, 59.9114) -> (-32.7356, 59.7562) construction
  line L785 (-32.7356, 59.7562) -> (-32.9401, 59.7421) construction
  spline S109 degree 3 poles (-32.9401, 59.7421) (-33.0319, 59.7351) (-33.1165, 59.7633) (-33.2152, 59.8057) knots 3 3 3 3 4 4 4 4
  line L786 (-32.9401, 59.7421) -> (-33.0319, 59.7351) construction
  line L787 (-33.0319, 59.7351) -> (-33.1165, 59.7633) construction
  line L788 (-33.1165, 59.7633) -> (-33.2152, 59.8057) construction
  line L789 (-33.2152, 59.8057) -> (-36.7777, 61.2871)
  spline S110 degree 3 poles (-36.7777, 61.2871) (-37.1727, 61.4423) (-37.3209, 61.6539) (-37.3209, 61.9713) knots 5 5 5 5 6 6 6 6
  line L790 (-36.7777, 61.2871) -> (-37.1727, 61.4423) construction
  line L791 (-37.1727, 61.4423) -> (-37.3209, 61.6539) construction
  line L792 (-37.3209, 61.6539) -> (-37.3209, 61.9713) construction
  line L793 (-37.3209, 61.9713) -> (-37.3209, 62.0207)
  spline S111 degree 3 poles (-37.3209, 62.0207) (-37.3209, 62.3452) (-37.1727, 62.5498) (-36.7777, 62.712) knots 7 7 7 7 8 8 8 8
  line L794 (-37.3209, 62.0207) -> (-37.3209, 62.3452) construction
  line L795 (-37.3209, 62.3452) -> (-37.1727, 62.5498) construction
  line L796 (-37.1727, 62.5498) -> (-36.7777, 62.712) construction
  line L797 (-36.7777, 62.712) -> (-33.1871, 64.1934)
  spline S112 degree 3 poles (-33.1871, 64.1934) (-33.0953, 64.2287) (-33.0178, 64.2499) (-32.9613, 64.2499) (-32.7427, 64.2499) (-32.5873, 64.0735) (-32.5873, 63.8407) (-32.5873, 63.6714) (-32.6932, 63.5303) (-32.8837, 63.4527) knots 9 9 9 9 10 10 10 11 11 11 12 12 12 12
  line L798 (-33.1871, 64.1934) -> (-33.0953, 64.2287) construction
  line L799 (-33.0953, 64.2287) -> (-33.0178, 64.2499) construction
  line L800 (-33.0178, 64.2499) -> (-32.9613, 64.2499) construction
  line L801 (-32.9613, 64.2499) -> (-32.7427, 64.2499) construction
  line L802 (-32.7427, 64.2499) -> (-32.5873, 64.0735) construction
  line L803 (-32.5873, 64.0735) -> (-32.5873, 63.8407) construction
  line L804 (-32.5873, 63.8407) -> (-32.5873, 63.6714) construction
  line L805 (-32.5873, 63.6714) -> (-32.6932, 63.5303) construction
  line L806 (-32.6932, 63.5303) -> (-32.8837, 63.4527) construction
  line L807 (-32.8837, 63.4527) -> (-33.7726, 63.093)
  line L808 (-33.7726, 63.093) -> (-33.7726, 60.8849)
  line L809 (-34.478, 62.8179) -> (-36.5448, 62.0066)
  line L810 (-36.5448, 62.0066) -> (-36.5448, 61.9855)
  line L811 (-36.5448, 61.9855) -> (-34.478, 61.1531)
  line L812 (-34.478, 61.1531) -> (-34.478, 62.8179)
  line L813 (-32.9754, 65.196) -> (-36.9471, 65.196)
  spline S113 degree 3 poles (-36.9471, 65.196) (-37.1515, 65.196) (-37.2785, 65.3229) (-37.2785, 65.5486) knots 1 1 1 1 2 2 2 2
  line L814 (-36.9471, 65.196) -> (-37.1515, 65.196) construction
  line L815 (-37.1515, 65.196) -> (-37.2785, 65.3229) construction
  line L816 (-37.2785, 65.3229) -> (-37.2785, 65.5486) construction
  line L817 (-37.2785, 65.5486) -> (-37.2785, 67.0511)
  spline S114 degree 3 poles (-37.2785, 67.0511) (-37.2785, 68.1799) (-36.7212, 68.7513) (-35.9594, 68.7513) (-35.4937, 68.7513) (-35.0917, 68.455) (-34.9365, 68.0742) knots 3 3 3 3 4 4 4 5 5 5 5
  line L818 (-37.2785, 67.0511) -> (-37.2785, 68.1799) construction
  line L819 (-37.2785, 68.1799) -> (-36.7212, 68.7513) construction
  line L820 (-36.7212, 68.7513) -> (-35.9594, 68.7513) construction
  line L821 (-35.9594, 68.7513) -> (-35.4937, 68.7513) construction
  line L822 (-35.4937, 68.7513) -> (-35.0917, 68.455) construction
  line L823 (-35.0917, 68.455) -> (-34.9365, 68.0742) construction
  spline S115 degree 3 poles (-34.9365, 68.0742) (-34.7672, 68.6102) (-34.3369, 68.8782) (-33.9066, 68.8782) (-33.18, 68.8782) (-32.6367, 68.2998) (-32.6367, 67.2346) knots 5 5 5 5 6 6 6 7 7 7 7
  line L824 (-34.9365, 68.0742) -> (-34.7672, 68.6102) construction
  line L825 (-34.7672, 68.6102) -> (-34.3369, 68.8782) construction
  line L826 (-34.3369, 68.8782) -> (-33.9066, 68.8782) construction
  line L827 (-33.9066, 68.8782) -> (-33.18, 68.8782) construction
  line L828 (-33.18, 68.8782) -> (-32.6367, 68.2998) construction
  line L829 (-32.6367, 68.2998) -> (-32.6367, 67.2346) construction
  line L830 (-32.6367, 67.2346) -> (-32.6367, 65.5486)
  spline S116 degree 3 poles (-32.6367, 65.5486) (-32.6367, 65.3229) (-32.7637, 65.196) (-32.9754, 65.196) knots 8 8 8 8 9 9 9 9
  line L831 (-32.6367, 65.5486) -> (-32.6367, 65.3229) construction
  line L832 (-32.6367, 65.3229) -> (-32.7637, 65.196) construction
  line L833 (-32.7637, 65.196) -> (-32.9754, 65.196) construction
  spline S117 degree 3 poles (-35.2045, 67.1006) (-35.2045, 67.6156) (-35.4304, 67.947) (-35.8748, 67.947) (-36.3192, 67.947) (-36.566, 67.6086) (-36.566, 66.9948) knots 0 0 0 0 1 1 1 2 2 2 2
  line L834 (-35.2045, 67.1006) -> (-35.2045, 67.6156) construction
  line L835 (-35.2045, 67.6156) -> (-35.4304, 67.947) construction
  line L836 (-35.4304, 67.947) -> (-35.8748, 67.947) construction
  line L837 (-35.8748, 67.947) -> (-36.3192, 67.947) construction
  line L838 (-36.3192, 67.947) -> (-36.566, 67.6086) construction
  line L839 (-36.566, 67.6086) -> (-36.566, 66.9948) construction
  line L840 (-36.566, 66.9948) -> (-36.566, 66.113)
  spline S118 degree 3 poles (-36.566, 66.113) (-36.566, 66.0143) (-36.5237, 65.972) (-36.4038, 65.972) knots 3 3 3 3 4 4 4 4
  line L841 (-36.566, 66.113) -> (-36.566, 66.0143) construction
  line L842 (-36.566, 66.0143) -> (-36.5237, 65.972) construction
  line L843 (-36.5237, 65.972) -> (-36.4038, 65.972) construction
  line L844 (-36.4038, 65.972) -> (-35.2045, 65.972)
  line L845 (-35.2045, 65.972) -> (-35.2045, 67.1006)
  line L846 (-33.3562, 66.113) -> (-33.3562, 67.1641)
  spline S119 degree 3 poles (-33.3562, 67.1641) (-33.3562, 67.7918) (-33.575, 68.0671) (-33.9841, 68.0671) (-34.3157, 68.0671) (-34.5767, 67.806) (-34.5767, 67.2911) knots 1 1 1 1 2 2 2 3 3 3 3
  line L847 (-33.3562, 67.1641) -> (-33.3562, 67.7918) construction
  line L848 (-33.3562, 67.7918) -> (-33.575, 68.0671) construction
  line L849 (-33.575, 68.0671) -> (-33.9841, 68.0671) construction
  line L850 (-33.9841, 68.0671) -> (-34.3157, 68.0671) construction
  line L851 (-34.3157, 68.0671) -> (-34.5767, 67.806) construction
  line L852 (-34.5767, 67.806) -> (-34.5767, 67.2911) construction
  line L853 (-34.5767, 67.2911) -> (-34.5767, 65.972)
  line L854 (-34.5767, 65.972) -> (-33.5185, 65.972)
  spline S120 degree 3 poles (-33.5185, 65.972) (-33.3916, 65.972) (-33.3562, 66.0143) (-33.3562, 66.113) knots 5 5 5 5 6 6 6 6
  line L855 (-33.5185, 65.972) -> (-33.3916, 65.972) construction
  line L856 (-33.3916, 65.972) -> (-33.3562, 66.0143) construction
  line L857 (-33.3562, 66.0143) -> (-33.3562, 66.113) construction
  spline S121 degree 3 poles (-34.9648, 69.6269) (-36.3545, 69.6269) (-37.3562, 70.6992) (-37.3562, 72.0958) (-37.3562, 73.4926) (-36.3545, 74.572) (-34.9648, 74.572) (-33.5679, 74.572) (-32.5592, 73.4926) (-32.5592, 72.0958) (-32.5592, 70.6992) (-33.5679, 69.6269) (-34.9648, 69.6269) knots 0 0 0 0 1 1 1 2 2 2 3 3 3 4 4 4 4
  line L858 (-34.9648, 69.6269) -> (-36.3545, 69.6269) construction
  line L859 (-36.3545, 69.6269) -> (-37.3562, 70.6992) construction
  line L860 (-37.3562, 70.6992) -> (-37.3562, 72.0958) construction
  line L861 (-37.3562, 72.0958) -> (-37.3562, 73.4926) construction
  line L862 (-37.3562, 73.4926) -> (-36.3545, 74.572) construction
  line L863 (-36.3545, 74.572) -> (-34.9648, 74.572) construction
  line L864 (-34.9648, 74.572) -> (-33.5679, 74.572) construction
  line L865 (-33.5679, 74.572) -> (-32.5592, 73.4926) construction
  line L866 (-32.5592, 73.4926) -> (-32.5592, 72.0958) construction
  line L867 (-32.5592, 72.0958) -> (-32.5592, 70.6992) construction
  line L868 (-32.5592, 70.6992) -> (-33.5679, 69.6269) construction
  line L869 (-33.5679, 69.6269) -> (-34.9648, 69.6269) construction
  spline S122 degree 3 poles (-33.3211, 72.0958) (-33.3211, 72.9636) (-33.9419, 73.7253) (-34.9577, 73.7253) (-35.9735, 73.7253) (-36.5943, 72.9636) (-36.5943, 72.0958) (-36.5943, 71.2352) (-35.9735, 70.4733) (-34.9577, 70.4733) (-33.9419, 70.4733) (-33.3211, 71.2352) (-33.3211, 72.0958) knots 0 0 0 0 1 1 1 2 2 2 3 3 3 4 4 4 4
  line L870 (-33.3211, 72.0958) -> (-33.3211, 72.9636) construction
  line L871 (-33.3211, 72.9636) -> (-33.9419, 73.7253) construction
  line L872 (-33.9419, 73.7253) -> (-34.9577, 73.7253) construction
  line L873 (-34.9577, 73.7253) -> (-35.9735, 73.7253) construction
  line L874 (-35.9735, 73.7253) -> (-36.5943, 72.9636) construction
  line L875 (-36.5943, 72.9636) -> (-36.5943, 72.0958) construction
  line L876 (-36.5943, 72.0958) -> (-36.5943, 71.2352) construction
  line L877 (-36.5943, 71.2352) -> (-35.9735, 70.4733) construction
  line L878 (-35.9735, 70.4733) -> (-34.9577, 70.4733) construction
  line L879 (-34.9577, 70.4733) -> (-33.9419, 70.4733) construction
  line L880 (-33.9419, 70.4733) -> (-33.3211, 71.2352) construction
  line L881 (-33.3211, 71.2352) -> (-33.3211, 72.0958) construction
  line L882 (-34.3581, 78.0999) -> (-33.2363, 79.2216)
  spline S123 degree 3 poles (-33.2363, 79.2216) (-33.1518, 79.3133) (-33.067, 79.3556) (-32.9613, 79.3556) (-32.7778, 79.3556) (-32.5873, 79.1863) (-32.5873, 78.9607) (-32.5873, 78.8337) (-32.6438, 78.749) (-32.7356, 78.6644) knots 1 1 1 1 2 2 2 3 3 3 4 4 4 4
  line L883 (-33.2363, 79.2216) -> (-33.1518, 79.3133) construction
  line L884 (-33.1518, 79.3133) -> (-33.067, 79.3556) construction
  line L885 (-33.067, 79.3556) -> (-32.9613, 79.3556) construction
  line L886 (-32.9613, 79.3556) -> (-32.7778, 79.3556) construction
  line L887 (-32.7778, 79.3556) -> (-32.5873, 79.1863) construction
  line L888 (-32.5873, 79.1863) -> (-32.5873, 78.9607) construction
  line L889 (-32.5873, 78.9607) -> (-32.5873, 78.8337) construction
  line L890 (-32.5873, 78.8337) -> (-32.6438, 78.749) construction
  line L891 (-32.6438, 78.749) -> (-32.7356, 78.6644) construction
  line L892 (-32.7356, 78.6644) -> (-34.2523, 77.2111)
  line L893 (-34.2523, 77.2111) -> (-34.2523, 76.4211)
  line L894 (-34.2523, 76.4211) -> (-32.933, 76.4211)
  spline S124 degree 3 poles (-32.933, 76.4211) (-32.7215, 76.4211) (-32.5873, 76.2588) (-32.5873, 76.033) (-32.5873, 75.8074) (-32.7215, 75.6451) (-32.933, 75.6451) knots 7 7 7 7 8 8 8 9 9 9 9
  line L895 (-32.933, 76.4211) -> (-32.7215, 76.4211) construction
  line L896 (-32.7215, 76.4211) -> (-32.5873, 76.2588) construction
  line L897 (-32.5873, 76.2588) -> (-32.5873, 76.033) construction
  line L898 (-32.5873, 76.033) -> (-32.5873, 75.8074) construction
  line L899 (-32.5873, 75.8074) -> (-32.7215, 75.6451) construction
  line L900 (-32.7215, 75.6451) -> (-32.933, 75.6451) construction
  line L901 (-32.933, 75.6451) -> (-36.9471, 75.6451)
  spline S125 degree 3 poles (-36.9471, 75.6451) (-37.1515, 75.6451) (-37.2785, 75.7721) (-37.2785, 75.9977) knots 10 10 10 10 11 11 11 11
  line L902 (-36.9471, 75.6451) -> (-37.1515, 75.6451) construction
  line L903 (-37.1515, 75.6451) -> (-37.2785, 75.7721) construction
  line L904 (-37.2785, 75.7721) -> (-37.2785, 75.9977) construction
  line L905 (-37.2785, 75.9977) -> (-37.2785, 77.451)
  spline S126 degree 3 poles (-37.2785, 77.451) (-37.2785, 78.749) (-36.5731, 79.2921) (-35.8112, 79.2921) (-35.2398, 79.2921) (-34.5486, 78.9395) (-34.3581, 78.0999) knots 12 12 12 12 13 13 13 14 14 14 14
  line L906 (-37.2785, 77.451) -> (-37.2785, 78.749) construction
  line L907 (-37.2785, 78.749) -> (-36.5731, 79.2921) construction
  line L908 (-36.5731, 79.2921) -> (-35.8112, 79.2921) construction
  line L909 (-35.8112, 79.2921) -> (-35.2398, 79.2921) construction
  line L910 (-35.2398, 79.2921) -> (-34.5486, 78.9395) construction
  line L911 (-34.5486, 78.9395) -> (-34.3581, 78.0999) construction
  spline S127 degree 3 poles (-34.9506, 77.3945) (-34.9506, 78.1705) (-35.3174, 78.4456) (-35.7618, 78.4456) (-36.1993, 78.4456) (-36.566, 78.1705) (-36.566, 77.3945) knots 0 0 0 0 1 1 1 2 2 2 2
  line L912 (-34.9506, 77.3945) -> (-34.9506, 78.1705) construction
  line L913 (-34.9506, 78.1705) -> (-35.3174, 78.4456) construction
  line L914 (-35.3174, 78.4456) -> (-35.7618, 78.4456) construction
  line L915 (-35.7618, 78.4456) -> (-36.1993, 78.4456) construction
  line L916 (-36.1993, 78.4456) -> (-36.566, 78.1705) construction
  line L917 (-36.566, 78.1705) -> (-36.566, 77.3945) construction
  line L918 (-36.566, 77.3945) -> (-36.566, 76.5622)
  spline S128 degree 3 poles (-36.566, 76.5622) (-36.566, 76.4633) (-36.5237, 76.4211) (-36.4038, 76.4211) knots 3 3 3 3 4 4 4 4
  line L919 (-36.566, 76.5622) -> (-36.566, 76.4633) construction
  line L920 (-36.566, 76.4633) -> (-36.5237, 76.4211) construction
  line L921 (-36.5237, 76.4211) -> (-36.4038, 76.4211) construction
  line L922 (-36.4038, 76.4211) -> (-34.9506, 76.4211)
  line L923 (-34.9506, 76.4211) -> (-34.9506, 77.3945)
  line L924 (-33.7726, 81.1693) -> (-32.8767, 80.8026)
  spline S129 degree 3 poles (-32.8767, 80.8026) (-32.6862, 80.7249) (-32.5873, 80.605) (-32.5873, 80.4216) (-32.5873, 80.1959) (-32.7356, 80.0407) (-32.9401, 80.0266) knots 1 1 1 1 2 2 2 3 3 3 3
  line L925 (-32.8767, 80.8026) -> (-32.6862, 80.7249) construction
  line L926 (-32.6862, 80.7249) -> (-32.5873, 80.605) construction
  line L927 (-32.5873, 80.605) -> (-32.5873, 80.4216) construction
  line L928 (-32.5873, 80.4216) -> (-32.5873, 80.1959) construction
  line L929 (-32.5873, 80.1959) -> (-32.7356, 80.0407) construction
  line L930 (-32.7356, 80.0407) -> (-32.9401, 80.0266) construction
  spline S130 degree 3 poles (-32.9401, 80.0266) (-33.0319, 80.0195) (-33.1165, 80.0478) (-33.2152, 80.0901) knots 3 3 3 3 4 4 4 4
  line L931 (-32.9401, 80.0266) -> (-33.0319, 80.0195) construction
  line L932 (-33.0319, 80.0195) -> (-33.1165, 80.0478) construction
  line L933 (-33.1165, 80.0478) -> (-33.2152, 80.0901) construction
  line L934 (-33.2152, 80.0901) -> (-36.7777, 81.5715)
  spline S131 degree 3 poles (-36.7777, 81.5715) (-37.1727, 81.7267) (-37.3209, 81.9383) (-37.3209, 82.2557) knots 5 5 5 5 6 6 6 6
  line L935 (-36.7777, 81.5715) -> (-37.1727, 81.7267) construction
  line L936 (-37.1727, 81.7267) -> (-37.3209, 81.9383) construction
  line L937 (-37.3209, 81.9383) -> (-37.3209, 82.2557) construction
  line L938 (-37.3209, 82.2557) -> (-37.3209, 82.3052)
  spline S132 degree 3 poles (-37.3209, 82.3052) (-37.3209, 82.6297) (-37.1727, 82.8342) (-36.7777, 82.9964) knots 7 7 7 7 8 8 8 8
  line L939 (-37.3209, 82.3052) -> (-37.3209, 82.6297) construction
  line L940 (-37.3209, 82.6297) -> (-37.1727, 82.8342) construction
  line L941 (-37.1727, 82.8342) -> (-36.7777, 82.9964) construction
  line L942 (-36.7777, 82.9964) -> (-33.1871, 84.4778)
  spline S133 degree 3 poles (-33.1871, 84.4778) (-33.0953, 84.5131) (-33.0178, 84.5343) (-32.9613, 84.5343) (-32.7427, 84.5343) (-32.5873, 84.3579) (-32.5873, 84.1252) (-32.5873, 83.9559) (-32.6932, 83.8148) (-32.8837, 83.7371) knots 9 9 9 9 10 10 10 11 11 11 12 12 12 12
  line L943 (-33.1871, 84.4778) -> (-33.0953, 84.5131) construction
  line L944 (-33.0953, 84.5131) -> (-33.0178, 84.5343) construction
  line L945 (-33.0178, 84.5343) -> (-32.9613, 84.5343) construction
  line L946 (-32.9613, 84.5343) -> (-32.7427, 84.5343) construction
  line L947 (-32.7427, 84.5343) -> (-32.5873, 84.3579) construction